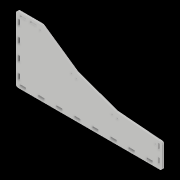
# Autodesk Inventor part: 9U Cheek V3
Saved by Autodesk Inventor 2018 (Build 220112000, 112)
## iProperties
Created: 2017-09-11
Part Number: 9U Cheek V3
Material: Generic
Document SubType Name: Modeling
Designer: gaine
Density: 1 g/cm^3
Appearance: Default
Author: gaine
Autodesk Inventor part; units mm, degrees
ref_plane "YZ Plane" through (0, 0, 0) normal (1, 0, 0) x (0, 1, 0)
ref_plane "XZ Plane" through (0, 0, 0) normal (0, 1, 0) x (-1, 0, 0)
ref_plane "XY Plane" through (0, 0, 0) normal (0, 0, 1) x (1, 0, 0)
sketch "Sketch1" plane through (0, 0, 0) normal (0, 0, 1) x (1, 0, 0)
  line L0 (447.8771, 77.149) -> (316.286, 87.8713)
  line L1 (314.6655, 88.2204) -> (190.8775, 132.4412)
  line L2 (189.4026, 133.1978) -> (82.2199, 207.2992)
  line L3 (0, 202.0759) -> (0, 6.35)
  circle A0 centre (440.5162, 61.8212) radius 2.413
  circle A1 centre (320.4926, 71.6009) radius 2.413
  line L4 (448.1345, 77.128) -> (443.7313, 23.0895) construction
  line L5 (315.4528, 87.9391) -> (312.3268, 49.5751) construction
  line L6 (315.4528, 87.9391) -> (300.5748, 46.291) construction
  circle A2 centre (190.7297, 115.6365) radius 2.413
  circle A3 centre (304.1324, 75.1256) radius 2.413
  line L7 (190.0903, 132.7224) -> (175.3821, 91.5497) construction
  line L8 (190.0903, 132.7224) -> (160.9674, 90.5981) construction
  circle A4 centre (175.8392, 123.2754) radius 2.413
  circle A5 centre (76.7856, 191.7567) radius 2.413
  line L9 (80.5901, 208.4259) -> (54.0448, 170.0299) construction
  line L10 (69.85, 208.4259) -> (76.2, 208.4259)
  line L11 (76.2, 202.0759) -> (76.2, 208.4259) construction
  line L12 (448.3928, 77.128) -> (454.4845, 77.128)
  line L13 (12.7, 208.4259) -> (6.35, 208.4259)
  line L14 (78.6088, 208.4259) -> (63.5, 208.4259)
  line L15 (12.7, 208.4259) -> (63.5, 208.4259)
  line L16 (12.7, 202.0759) -> (31.75, 202.0759)
  line L17 (31.75, 202.0759) -> (31.75, 195.7259)
  line L18 (31.75, 195.7259) -> (12.7, 195.7259)
  line L19 (12.7, 195.7259) -> (12.7, 202.0759)
  line L20 (44.45, 202.0759) -> (63.5, 202.0759)
  line L21 (63.5, 202.0759) -> (63.5, 195.7259)
  line L22 (63.5, 195.7259) -> (44.45, 195.7259)
  line L23 (44.45, 195.7259) -> (44.45, 202.0759)
  line L24 (63.5, 195.7259) -> (71.8099, 195.7259) construction
  line L25 (71.8099, 195.7259) -> (71.8099, 208.4259) construction
  line L26 (12.7, 6.35) -> (31.75, 6.35)
  line L27 (31.75, 6.35) -> (31.75, 12.7)
  line L28 (31.75, 12.7) -> (12.7, 12.7)
  line L29 (12.7, 12.7) -> (12.7, 6.35)
  line L30 (69.85, 12.7) -> (88.9, 12.7)
  line L31 (88.9, 12.7) -> (88.9, 6.35)
  line L32 (88.9, 6.35) -> (69.85, 6.35)
  line L33 (69.85, 6.35) -> (69.85, 12.7)
  line L34 (127, 12.7) -> (146.05, 12.7)
  line L35 (146.05, 12.7) -> (146.05, 6.35)
  line L36 (146.05, 6.35) -> (127, 6.35)
  line L37 (127, 6.35) -> (127, 12.7)
  line L38 (184.15, 12.7) -> (203.2, 12.7)
  line L39 (203.2, 12.7) -> (203.2, 6.35)
  line L40 (203.2, 6.35) -> (184.15, 6.35)
  line L41 (184.15, 6.35) -> (184.15, 12.7)
  line L42 (241.3, 12.7) -> (260.35, 12.7)
  line L43 (260.35, 12.7) -> (260.35, 6.35)
  line L44 (260.35, 6.35) -> (241.3, 6.35)
  line L45 (241.3, 6.35) -> (241.3, 12.7)
  line L46 (298.45, 12.7) -> (317.5, 12.7)
  line L47 (317.5, 12.7) -> (317.5, 6.35)
  line L48 (317.5, 6.35) -> (298.45, 6.35)
  line L49 (298.45, 6.35) -> (298.45, 12.7)
  line L50 (355.6, 12.7) -> (374.65, 12.7)
  line L51 (374.65, 12.7) -> (374.65, 6.35)
  line L52 (374.65, 6.35) -> (355.6, 6.35)
  line L53 (355.6, 6.35) -> (355.6, 12.7)
  line L54 (412.75, 12.7) -> (431.8, 12.7)
  line L55 (431.8, 12.7) -> (431.8, 6.35)
  line L56 (431.8, 6.35) -> (412.75, 6.35)
  line L57 (412.75, 6.35) -> (412.75, 12.7)
  line L58 (460.8345, 70.778) -> (460.8345, 6.35)
  line L59 (454.4845, 0) -> (454.4845, 0)
  line L60 (448.1345, 12.7) -> (454.4845, 12.7)
  line L61 (454.4845, 12.7) -> (454.4845, 31.75)
  line L62 (454.4845, 31.75) -> (448.1345, 31.75)
  line L63 (448.1345, 31.75) -> (448.1345, 12.7)
  line L64 (448.1345, 51.728) -> (454.4845, 51.728)
  line L65 (454.4845, 51.728) -> (454.4845, 70.778)
  line L66 (454.4845, 70.778) -> (448.1345, 70.778)
  line L67 (448.1345, 70.778) -> (448.1345, 51.728)
  line L68 (6.35, 189.3759) -> (12.7, 189.3759)
  line L69 (12.7, 189.3759) -> (12.7, 170.3259)
  line L70 (12.7, 170.3259) -> (6.35, 170.3259)
  line L71 (6.35, 170.3259) -> (6.35, 189.3759)
  line L72 (6.35, 139.8459) -> (12.7, 139.8459)
  line L73 (12.7, 139.8459) -> (12.7, 120.7959)
  line L74 (12.7, 120.7959) -> (6.35, 120.7959)
  line L75 (6.35, 120.7959) -> (6.35, 139.8459)
  line L76 (6.35, 90.3159) -> (12.7, 90.3159)
  line L77 (12.7, 90.3159) -> (12.7, 71.2659)
  line L78 (12.7, 71.2659) -> (6.35, 71.2659)
  line L79 (6.35, 71.2659) -> (6.35, 90.3159)
  line L80 (6.35, 40.7859) -> (12.7, 40.7859)
  line L81 (12.7, 40.7859) -> (12.7, 21.7359)
  line L82 (12.7, 21.7359) -> (6.35, 21.7359)
  line L83 (6.35, 21.7359) -> (6.35, 40.7859)
  arc A6 (6.35, 208.4259) -> (0, 202.0759) centre (6.35, 202.0759) ccw
  arc A7 (82.2199, 207.2992) -> (78.6088, 208.4259) centre (78.6088, 202.0759) ccw
  arc A8 (189.4026, 133.1978) -> (190.8775, 132.4412) centre (193.0137, 138.4211) ccw
  arc A9 (314.6655, 88.2204) -> (316.286, 87.8713) centre (316.8017, 94.2003) ccw
  arc A10 (447.8771, 77.149) -> (448.3928, 77.128) centre (448.3928, 83.478) ccw
  arc A11 (460.8345, 70.778) -> (454.4845, 77.128) centre (454.4845, 70.778) ccw
  arc A12 (454.4845, 0) -> (460.8345, 6.35) centre (454.4845, 6.35) ccw
  arc A13 (0, 6.35) -> (6.35, 0) centre (6.35, 6.35) ccw
  line L84 (6.35, 0) -> (454.4845, 0)
  point P0 (0, 0)
  point P1 (0, 0)
  point P2 (460.8345, 77.128)
  dimension "d3" = 4.826
  dimension "d4" = 4.826
  dimension "d5" = 15.875
  dimension "d6" = 15.875
  dimension "d7" = 120.4214
  dimension "d8" = 90
  dimension "d9" = 6.35
  dimension "d11" = 90
  dimension "d12" = 90
  dimension "d13" = 165
  dimension "d14" = 6.35
  dimension "d16" = 4.826
  dimension "d17" = 4.826
  dimension "d18" = 6.35
  dimension "d19" = 15.875
  dimension "d20" = 15.875
  dimension "d21" = 120.4214
  dimension "d22" = 165
  dimension "d23" = 90
  dimension "d24" = 90
  dimension "d25" = 6.35
  dimension "d26" = 4.826
  dimension "d27" = 4.826
  dimension "d28" = 6.35
  dimension "d29" = 15.875
  dimension "d30" = 15.875
  dimension "d31" = 120.4214
  dimension "d32" = 90
  dimension "d33" = 6.35
  dimension "d38" = 6.35
  dimension "d39" = 12.7
  dimension "d41" = 76.2
  dimension "d76" = 19.05
  dimension "d77" = 6.35
  dimension "d78" = 19.05
  dimension "d79" = 6.35
  dimension "d80" = 12.7
  dimension "d81" = 12.7
  dimension "d82" = 6.35
  dimension "d83" = 6.35
  dimension "d84" = 71.8099
  dimension "d86" = 6.35
  dimension "d87" = 19.05
  dimension "d88" = 6.35
  dimension "d89" = 19.05
  dimension "d91" = 6.35
  dimension "d92" = 6.35
  dimension "d93" = 6.35
  dimension "d94" = 6.35
  dimension "d97" = 19.05
  dimension "d98" = 19.05
  dimension "d99" = 19.05
  dimension "d100" = 19.05
  dimension "d102" = 12.7
  dimension "d106" = 38.1
  dimension "d107" = 38.1
  dimension "d109" = 38.1
  dimension "d112" = 38.1
  dimension "d113" = 38.1
  dimension "d115" = 19.05
  dimension "d116" = 6.35
  dimension "d117" = 38.1
  dimension "d119" = 38.1
  dimension "d120" = 6.35
  constraints: 170 end point, 32 parallel, 24 horizontal, 19 perpendicular, 17 point on line, 16 point on circle, 16 tangent, 14 centre point, 7 equal radius, 1 coincident, 1 vertical
  measures "d3" diameter of A0
  measures "d4" diameter of A1
  measures "d5" distance from line of L0 A1.centre
  measures "d6" distance from line of L0 A0.centre
  measures "d7" distance of A0.centre A1.centre
  measures "d8" angle of L4 L0
  measures "d9" distance from line of L4 A0.centre
  measures "d11" angle of L6 L1
  measures "d12" angle of L0 L5
  measures "d13" angle of L0 L1
  measures "d14" distance from line of L5 A1.centre
  measures "d16" diameter of A3
  measures "d17" diameter of A2
  measures "d18" distance from line of L6 A3.centre
  measures "d19" distance from line of L1 A3.centre
  measures "d20" distance from line of L1 A2.centre
  measures "d21" distance of A3.centre A2.centre
  measures "d22" angle of L1 L2
  measures "d23" angle of L1 L7
  measures "d24" angle of L2 L8
  measures "d25" distance from line of A2.centre L7
  measures "d26" diameter of A5
  measures "d27" diameter of A4
  measures "d28" distance from line of L8 A4.centre
  measures "d29" distance from line of L2 A4.centre
  measures "d30" distance from line of L2 A5.centre
  measures "d31" distance of A4.centre A5.centre
  measures "d32" angle of L2 L9
  measures "d33" distance from line of L9 A5.centre
  measures "d38" distance of L10.end L11.start
  measures "d39" distance of L4.start point (460.834, 77.128)
  measures "d41" distance between parallel lines of L3 L11
  measures "d76" distance of L17.end L18.end
  measures "d77" distance of L16.end L17.end
  measures "d78" distance of L21.end L22.end
  measures "d79" distance of L20.end L21.end
  measures "d80" distance between parallel lines of L3 L19
  measures "d81" distance between parallel lines of L17 L23
  measures "d82" distance between parallel lines of L15 L16
  measures "d83" distance between parallel lines of L20 L15
  measures "d84" distance between parallel lines of L25 L3
  measures "d86" distance of L26.end L27.end
  measures "d87" distance of L26.start L26.end
  measures "d88" distance of L30.end L31.end
  measures "d89" distance of L31.end L32.end
  measures "d91" distance of L34.end L35.end
  measures "d92" distance of L38.end L39.end
  measures "d93" distance of L42.end L43.end
  measures "d94" distance of L46.end L47.end
  measures "d97" distance of L46.start L46.end
  measures "d98" distance of L42.start L42.end
  measures "d99" distance of L38.start L38.end
  measures "d100" distance of L34.start L34.end
  measures "d102" distance between parallel lines of L3 L29
  measures "d106" distance between parallel lines of L33 L27
  measures "d107" distance between parallel lines of L31 L37
  measures "d109" distance between parallel lines of L35 L41
  measures "d112" distance between parallel lines of L39 L45
  measures "d113" distance between parallel lines of L43 L49
  measures "d115" distance of L51.end L52.end
  measures "d116" distance of L50.end L51.end
  measures "d117" distance between parallel lines of L53 L47
  measures "d119" distance between parallel lines of L51 L57
  measures "d120" distance between parallel lines of L56 L54
extrude "Extrusion2" add sketch "Sketch1" along normal blind 6.35
equation "\"d4\" = d3"
equation "\"d5\" = d6"
equation "\"d14\" = d9"
equation "\"d16\" = d3"
equation "\"d17\" = d3"
equation "\"d18\" = d9"
equation "\"d19\" = d6"
equation "\"d20\" = d6"
equation "\"d21\" = d7"
equation "\"d22\" = d13"
equation "\"d25\" = d9"
equation "\"d26\" = d3"
equation "\"d27\" = d3"
equation "\"d28\" = d9"
equation "\"d29\" = d6"
equation "\"d30\" = d6"
equation "\"d31\" = d7"
equation "\"d33\" = d9"
equation "\"d78\" = d76"
equation "\"d81\" = d80"
equation "\"d83\" = d82"
equation "\"d86\" = d77"
equation "\"d87\" = d76"
equation "\"d88\" = d86"
equation "\"d89\" = d87"
equation "\"d91\" = d86"
equation "\"d92\" = d86"
equation "\"d93\" = d86"
equation "\"d94\" = d93"
body "Solid2"
